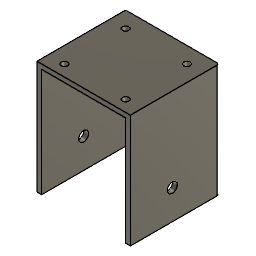
Motor Bracket (Autodesk Fusion 360 design; units mm, degrees)
part number: 2026-05-02-17-38-57-581
Autodesk Fusion 360 part; units mm, degrees
sketch "Sketch1" plane through (0, 0, 0) normal (0, 0, 1) x (1, 0, 0)
  line L0 (-1.731, 4) -> (40.819, 4)
  line L1 (40.819, 4) -> (40.819, -38.55)
  line L2 (40.819, -38.55) -> (-1.731, -38.55)
  line L3 (-1.731, -38.55) -> (-1.731, 4)
  line L4 (-1.731, -38.55) -> (-4.131, -38.55)
  line L5 (-4.131, -38.55) -> (-4.131, 4)
  line L6 (-4.131, 4) -> (-1.731, 4)
  line L7 (-1.731, 4) -> (-1.731, -38.55)
  line L8 (-4.131, 4) -> (40.819, 4)
  line L9 (40.819, 4) -> (40.819, 6.4)
  line L10 (40.819, 6.4) -> (-4.131, 6.4)
  line L11 (-4.131, 6.4) -> (-4.131, 4)
  line L12 (40.819, -38.55) -> (43.219, -38.55)
  line L13 (43.219, -38.55) -> (43.219, 6.4)
  line L14 (43.219, 6.4) -> (40.819, 6.4)
  line L15 (40.819, 6.4) -> (40.819, -38.55)
  circle A0 centre (4.044, -1.775) radius 1.625
  circle A1 centre (35.044, -1.775) radius 1.625
  circle A2 centre (4.044, -32.775) radius 1.625
  circle A3 centre (35.044, -32.775) radius 1.625
  dimension "d1" = 42.55
  dimension "d2" = 42.55
  dimension "d3" = 2.4
  dimension "d4" = 2.4
  dimension "d5" = 2.4
  dimension "d6" = 44.95
  dimension "d7" = 3.25
  dimension "d8" = 3.25
  dimension "d9" = 3.25
  dimension "d10" = 3.25
  dimension "d11" = 31
  dimension "d12" = 31
  dimension "d13" = 31
  dimension "d14" = 5.775
  dimension "d15" = 5.775
  constraint horizontal L0
  constraint vertical L1
  constraint horizontal L2
  constraint vertical L3
  constraint horizontal L4
  constraint vertical L5
  constraint horizontal L6
  constraint vertical L7
  constraint horizontal L8
  constraint vertical L9
  constraint horizontal L10
  constraint vertical L11
  constraint horizontal L12
  constraint vertical L13
  constraint horizontal L14
  constraint vertical L15
  measures "d1" distance of L0.start L2.end
  measures "d2" distance of L1 L3
  measures "d3" distance of L3 L5
  measures "d4" distance of L5.end L10.end
  measures "d5" distance of L13 L15
  measures "d6" distance of L9 L11
  measures "d7" diameter of A0
  measures "d8" diameter of A1
  measures "d9" diameter of A2
  measures "d10" diameter of A3
  measures "d11" distance of A0.centre A1.centre
  measures "d12" distance of A2.centre A3.centre
  measures "d13" distance of A0.centre A2.centre
  measures "d14" distance of L3 A0.centre
  measures "d15" distance of L0 A0.centre
extrude "Extrude1" add sketch "Sketch1" along normal blind 2.4 contours L0 L6 L8 L9 L10 L11 L15 | L0 L1 L2 L3 L7 L8 L15 | L3 L4 L5 L6 L7 L8 makes body 1
extrude "Extrude2" add sketch "Sketch1" against normal blind 34.25 separate body contours L0 L6 L8 L9 L10 L11 L15 | L3 L4 L5 L6 L7 L8 | L1 L9 L12 L13 L14 L15 makes body 2
extrude "Extrude3" add 1 faces at (42.419, -9.3833, 0) along direction (0, 0, 1) blind 2.4 on bodies 2 bodies 1 2
fillet "Fillet1" radius 1 1 edges at (-4.131, 6.4, -15.925) on bodies 1
fillet "Fillet2" radius 1 1 edges at (43.219, 6.4, -15.925) on bodies 1
extrude "Extrude4" add 1 faces at (26.6357, 5.6, -34.25) along direction (0, 0, -1) blind 20.75 on bodies 1 bodies 1
sketch "Sketch2" plane through (0, 4, 0) normal (0, -1, 0) x (1, 0, 0)
  line L0 (40.819, 0) -> (-1.731, 0)
  line L1 (-1.731, 0) -> (-1.731, -55)
  line L2 (-1.731, -55) -> (40.819, -55)
  line L3 (40.819, -55) -> (40.819, 0)
  circle A0 centre (19.544, -15) radius 2.5
  dimension "d28" = 5
  dimension "d29" = 15
  dimension "d30" = 21.275
  measures "d28" diameter of A0
  measures "d29" distance of L0 A0.centre
  measures "d30" distance of L1 A0.centre
extrude "Extrude5" cut sketch "Sketch2" against normal blind 2.4 contours A0 bodies 1
sketch "Sketch3" plane through (-1.731, 0, 0) normal (1, 0, 0) x (0, 1, 0)
  line L0 (4, 0) -> (-38.55, 0)
  line L1 (-38.55, 0) -> (-38.55, -55)
  line L2 (-38.55, -55) -> (4, -55)
  line L3 (4, -55) -> (4, 0)
  circle A0 centre (-17.275, -40) radius 2.5
  dimension "d33" = 5
  dimension "d34" = 40
  dimension "d35" = 21.275
  measures "d33" diameter of A0
  measures "d34" distance of L0 A0.centre
  measures "d35" distance of L1 A0.centre
extrude "Extrude6" cut sketch "Sketch3" against normal blind 2.4 contours A0 bodies 1
extrude "Extrude7" cut sketch "Sketch3" along normal blind 72 contours A0 bodies 1
